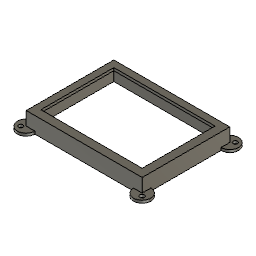
FullBoxDispenser_Assembly (Autodesk Fusion 360 archive; units mm, degrees)
design "BasicBreadboardHolder"
part number: 2026-05-25-11-22-07-482
Autodesk Fusion 360 part; units mm, degrees
note: some values were not read from the file. Set by a fixed rule: which sketch regions a step uses.
sketch "Sketch1" plane through (0, 0, 0) normal (0, 0, 1) x (1, 0, 0)
  line L0 (0, 0) -> (82, 0)
  line L1 (82, 0) -> (82, 61)
  line L2 (82, 61) -> (0, 61)
  line L3 (0, 61) -> (0, 0)
  line L4 (-2, 63) -> (84, 63)
  line L5 (84, 63) -> (84, -2)
  line L6 (84, -2) -> (-2, -2)
  line L7 (-2, -2) -> (-2, 63)
  circle A0 centre (-2, -2) radius 6.5
  circle A1 centre (-2, 63) radius 6.5
  circle A2 centre (84, 63) radius 6.5
  circle A3 centre (84, -2) radius 6.5
  circle A4 centre (-4, -4) radius 1.65
  circle A5 centre (-4, 65) radius 1.65
  circle A6 centre (86, 65) radius 1.65
  circle A7 centre (86, -4) radius 1.65
  line L8 (3, 58) -> (78, 58)
  line L9 (78, 58) -> (78, 4)
  line L10 (78, 4) -> (3, 4)
  line L11 (3, 4) -> (3, 58)
  dimension "d1" = 61
  dimension "d2" = 82
  dimension "d3" = 2
  dimension "d4" = 2
  dimension "d5" = 2
  dimension "d6" = 2
  dimension "d7" = 13
  dimension "d8" = 13
  dimension "d9" = 13
  dimension "d10" = 13
  dimension "d11" = 3.3
  dimension "d12" = 2
  dimension "d13" = 2
  dimension "d14" = 3.3
  dimension "d15" = 2
  dimension "d16" = 2
  dimension "d17" = 3.3
  dimension "d18" = 2
  dimension "d19" = 2
  dimension "d20" = 3.3
  dimension "d21" = 2
  dimension "d22" = 2
  dimension "d23" = 3
  dimension "d24" = 4
  dimension "d25" = 3
  dimension "d26" = 4
  constraint horizontal L0
  constraint vertical L1
  constraint horizontal L2
  constraint vertical L3
  constraint coincident L0.start L3.end
  constraint horizontal L4
  constraint vertical L5
  constraint horizontal L6
  constraint vertical L7
  constraint coincident L6.end L7.start
  constraint coincident L4.start L7.end
  constraint coincident L4.end L5.start
  constraint coincident L5.end L6.start
  constraint horizontal L8
  constraint vertical L9
  constraint horizontal L10
  constraint vertical L11
  measures "d1" distance of L0.start L2.end
  measures "d2" distance of L0.start L0.end
  measures "d3" distance of L2 L4
  measures "d4" distance of L1 L5
  measures "d5" distance of L3 L7
  measures "d6" distance of L0 L6
  measures "d7" diameter of A0
  measures "d8" diameter of A1
  measures "d9" diameter of A2
  measures "d10" diameter of A3
  measures "d11" diameter of A4
  measures "d12" vertical distance of L6.end A4.centre
  measures "d13" horizontal distance of L6.end A4.centre
  measures "d14" diameter of A5
  measures "d15" vertical distance of L4.start A5.centre
  measures "d16" horizontal distance of L4.start A5.centre
  measures "d17" diameter of A6
  measures "d18" horizontal distance of L4.end A6.centre
  measures "d19" vertical distance of L4.end A6.centre
  measures "d20" diameter of A7
  measures "d21" horizontal distance of L5.end A7.centre
  measures "d22" vertical distance of L5.end A7.centre
  measures "d23" distance of L2 L8
  measures "d24" distance of L0 L10
  measures "d25" distance of L3 L11
  measures "d26" distance of L1 L9
extrude "Extrude1" add sketch "Sketch1" along normal blind 2 contours L6 L7 A0 | L5 L6 A3 | L4 L7 A1 | L4 L5 A2 makes body 1 at (85.5519, 61.1596, 2) makes body 2 at (85.5519, -0.1596, 0) makes body 3 at (-3.5519, 61.1596, 0) makes body 4 at (-3.5519, -0.1596, 0)
extrude "Extrude2" add sketch "Sketch1" along normal blind 10 contours L0 L3 L6 L7 A0 | L0 L6 A0 A3 | L3 L7 A0 A1 | L0 L1 L5 L6 A3 | L2 L3 L4 L7 A1 | L1 L5 A2 A3 | L2 L4 A1 A2 | L1 L2 L4 L5 A2 bodies 1 2 3 4
extrude "Extrude3" add sketch "Sketch1" along normal blind 2 from surface at 10 contours L0 L3 A0 | L0 L3 L6 L7 A0 | L0 L1 L2 L3 A0 A1 A2 A3 | L0 L6 A0 A3 | L3 L7 A0 A1 | L0 L1 A3 | L0 L1 L5 L6 A3 | L2 L3 L4 L7 A1 | L2 L3 A1 | L1 L5 A2 A3 | L2 L4 A1 A2 | L1 L2 A2 | L1 L2 L4 L5 A2 bodies 1

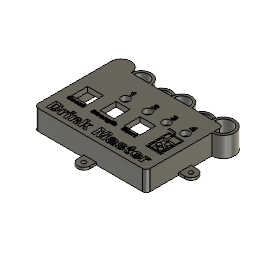
design "UIHolder"
part number: 2026-05-20-16-52-47-232
Autodesk Fusion 360 part; units mm, degrees
sketch "Sketch1" plane through (0, 0, 0) normal (0, 0, 1) x (1, 0, 0)
  line L0 (0, 0) -> (0, 57)
  line L1 (0, 0) -> (85, 0)
  line L2 (0, 57) -> (85, 57)
  line L3 (85, 57) -> (85, 0)
  line L4 (-2, 59) -> (87, 59)
  line L5 (87, 59) -> (87, -2)
  line L6 (87, -2) -> (-2, -2)
  line L7 (-2, -2) -> (-2, 59)
  circle A0 centre (6, 59) radius 6
  circle A1 centre (6, 59) radius 8
  line L8 (0, 59) -> (0, 57)
  line L9 (12, 59) -> (12, 57)
  circle A2 centre (77, 39) radius 3.25
  circle A3 centre (62, 39) radius 3.25
  circle A4 centre (47, 39) radius 3.25
  circle A5 centre (29.5, 39) radius 3.25
  line L10 (47.5, 32.5) -> (60, 32.5)
  line L11 (60, 32.5) -> (60, 20)
  line L12 (60, 20) -> (47.5, 20)
  line L13 (47.5, 20) -> (47.5, 32.5)
  line L14 (6, 20) -> (18.5, 20)
  line L15 (18.5, 20) -> (18.5, 32.5)
  line L16 (18.5, 32.5) -> (6, 32.5)
  line L17 (6, 32.5) -> (6, 20)
  line L18 (27.5, 33.5) -> (38.5, 33.5)
  line L19 (38.5, 33.5) -> (38.5, 21)
  line L20 (38.5, 21) -> (27.5, 21)
  line L21 (27.5, 21) -> (27.5, 33.5)
  circle A6 centre (22, 59) radius 8
  circle A7 centre (22, 59) radius 6
  circle A8 centre (38, 59) radius 8
  circle A9 centre (38, 59) radius 6
  circle A10 centre (54, 59) radius 8
  circle A11 centre (54, 59) radius 6
  circle A12 centre (70, 59) radius 8
  circle A13 centre (70, 59) radius 6
  circle A14 centre (87, 59) radius 9
  circle A15 centre (87, 59) radius 7
  circle A16 centre (-7, 28.5) radius 1.65
  circle A17 centre (42.5, -7) radius 1.65
  circle A18 centre (92, 28.5) radius 1.65
  line L22 (-2, 23.5) -> (-12, 23.5)
  line L23 (-12, 23.5) -> (-12, 33.5)
  line L24 (-12, 33.5) -> (-2, 33.5)
  line L25 (-2, 33.5) -> (-2, 23.5)
  line L26 (-2, 23.5) -> (-12, 33.5) construction
  line L27 (-12, 23.5) -> (-2, 33.5) construction
  line L28 (47.5, -2) -> (37.5, -2)
  line L29 (37.5, -2) -> (37.5, -12)
  line L30 (37.5, -12) -> (47.5, -12)
  line L31 (47.5, -12) -> (47.5, -2)
  line L32 (47.5, -2) -> (37.5, -12) construction
  line L33 (37.5, -2) -> (47.5, -12) construction
  line L34 (87, 23.5) -> (97, 23.5)
  line L35 (97, 23.5) -> (97, 33.5)
  line L36 (97, 33.5) -> (87, 33.5)
  line L37 (87, 33.5) -> (87, 23.5)
  line L38 (87, 23.5) -> (97, 33.5) construction
  line L39 (97, 23.5) -> (87, 33.5) construction
  point P0 (-7, 28.5)
  point P1 (42.5, -7)
  point P2 (92, 28.5)
  dimension "d1" = 57
  dimension "d2" = 85
  dimension "d3" = 85
  dimension "d4" = 2
  dimension "d5" = 2
  dimension "d6" = 2
  dimension "d7" = 2
  dimension "d8" = 12
  dimension "d9" = 8
  dimension "d12" = 6.5
  dimension "d13" = 8
  dimension "d15" = 6.5
  dimension "d17" = 15
  dimension "d18" = 6.5
  dimension "d20" = 15
  dimension "d21" = 6.5
  dimension "d22" = 18
  dimension "d23" = 18
  dimension "d24" = 18
  dimension "d25" = 18
  dimension "d26" = 17.5
  dimension "d27" = 12.5
  dimension "d28" = 12.5
  dimension "d29" = 25
  dimension "d30" = 20
  dimension "d31" = 12.5
  dimension "d32" = 12.5
  dimension "d33" = 20
  dimension "d34" = 6
  dimension "d35" = 12.5
  dimension "d36" = 11
  dimension "d37" = 9
  dimension "d38" = 21
  dimension "d42" = 16
  dimension "d43" = 12
  dimension "d44" = 16
  dimension "d45" = 12
  dimension "d46" = 16
  dimension "d47" = 12
  dimension "d48" = 16
  dimension "d49" = 12
  dimension "d50" = 14
  dimension "d75" = 3.3
  dimension "d76" = 3.3
  dimension "d77" = 3.3
  dimension "d78" = 30.5
  dimension "d79" = 30.5
  dimension "d80" = 44.5
  dimension "d81" = 5
  dimension "d82" = 5
  dimension "d83" = 5
  dimension "d84" = 10
  dimension "d85" = 10
  dimension "d86" = 10
  dimension "d87" = 10
  dimension "d88" = 10
  dimension "d89" = 10
  constraint coincident L0.start L1.start
  constraint vertical L0
  constraint perpendicular L0 L1
  constraint perpendicular L0 L2
  constraint horizontal L4
  constraint vertical L5
  constraint horizontal L6
  constraint vertical L7
  constraint coincident L4 A0.centre
  constraint concentric A0 A1
  constraint coincident L4.start A1
  constraint coincident A0 L8.start
  constraint coincident L4 L8.start
  constraint coincident L4 L9.start
  constraint coincident A0 L9.start
  constraint coincident L2 L9.end
  constraint perpendicular L2 L9
  constraint horizontal L10
  constraint vertical L11
  constraint horizontal L12
  constraint vertical L13
  constraint horizontal L14
  constraint vertical L15
  constraint horizontal L16
  constraint vertical L17
  constraint horizontal L18
  constraint vertical L19
  constraint horizontal L20
  constraint vertical L21
  constraint coincident L4 A6.centre
  constraint tangent A1 A6
  constraint concentric A6 A7
  constraint coincident L4 A8.centre
  constraint tangent A6 A8
  constraint concentric A8 A9
  constraint coincident L4 A10.centre
  constraint tangent A8 A10
  constraint concentric A10 A11
  constraint coincident L4 A12.centre
  constraint tangent A10 A12
  constraint concentric A12 A13
  constraint coincident L4.end L5.start
  constraint tangent A12 A14
  constraint concentric A14 A15
  constraint horizontal L22
  constraint perpendicular L22 L23
  constraint parallel L22 L24
  constraint parallel L23 L25
  constraint coincident L26 P0
  constraint coincident L27 P0
  constraint coincident P0 A16.centre
  constraint horizontal L28
  constraint perpendicular L28 L29
  constraint parallel L28 L30
  constraint parallel L29 L31
  constraint coincident L32 P1
  constraint coincident L33 P1
  constraint coincident P1 A17.centre
  constraint horizontal L34
  constraint perpendicular L34 L35
  constraint parallel L34 L36
  constraint parallel L35 L37
  constraint coincident L38 P2
  constraint coincident L39 P2
  constraint coincident P2 A18.centre
  measures "d1" distance of L0.start L0.end
  measures "d2" distance of L0.start L1.end
  measures "d3" distance of L0.end L2.end
  measures "d4" distance of L2 L4
  measures "d5" distance of L0 L7
  measures "d6" distance of L1 L6
  measures "d7" distance of L3 L5
  measures "d8" diameter of A0
  measures "d9" distance of L4.start A0.centre
  measures "d12" diameter of A2
  measures "d13" distance of L3 A2.centre
  measures "d15" diameter of A3
  measures "d17" distance of A2.centre A3.centre
  measures "d18" diameter of A4
  measures "d20" distance of A3.centre A4.centre
  measures "d21" diameter of A5
  measures "d22" distance of L2 A5.centre
  measures "d23" distance of L2 A4.centre
  measures "d24" distance of L2 A3.centre
  measures "d25" distance of L2 A2.centre
  measures "d26" distance of A4.centre A5.centre
  measures "d27" distance of L10.start L10.end
  measures "d28" distance of L10.start L12.end
  measures "d29" distance of L3 L11
  measures "d30" distance of L1 L12
  measures "d31" distance of L15.end L16.end
  measures "d32" distance of L14.end L15.end
  measures "d33" distance of L1 L14
  measures "d34" distance of L0 L17
  measures "d35" distance of L18.start L20.end
  measures "d36" distance of L18.start L18.end
  measures "d37" distance of L13 L19
  measures "d38" distance of L1 L20
  measures "d42" diameter of A6
  measures "d43" diameter of A7
  measures "d44" diameter of A8
  measures "d45" diameter of A9
  measures "d46" diameter of A10
  measures "d47" diameter of A11
  measures "d48" diameter of A12
  measures "d49" diameter of A13
  measures "d50" diameter of A15
  measures "d75" diameter of A16
  measures "d76" diameter of A17
  measures "d77" diameter of A18
  measures "d78" vertical distance of L4.start P0
  measures "d79" vertical distance of L4.end P2
  measures "d80" horizontal distance of L5.end P1
  measures "d81" distance of L6 P1
  measures "d82" distance of L7 P0
  measures "d83" distance of L5 P2
  measures "d84" distance of L22.end L23.end
  measures "d85" distance of L22.start L22.end
  measures "d86" distance of L29.end L30.end
  measures "d87" distance of L28.start L30.end
  measures "d88" distance of L34.end L35.end
  measures "d89" distance of L35.end L36.end
extrude "Extrude4" add sketch "Sketch1" along normal blind 2 contours L7 L22 L23 L24 L25 | L5 L34 L35 L36 L37 | L6 L28 L29 L30 L31 makes body 1 at (-7.0411, 24.6182, 0) makes body 2 at (42.5411, -3.1182, 0) makes body 3 at (91.9589, 24.6182, 0)
fillet "Fillet4" radius 5 6 edges at (-12, 23.5, 1) (-12, 33.5, 1) (37.5, -12, 1) (47.5, -12, 1) (97, 23.5, 1) (97, 33.5, 1) on bodies 1 2 3
extrude "Extrude1" add sketch "Sketch1" along normal blind 12 contours L0 L1 L3 L5 L6 L7 A1 A14 L25 L28 L37 | L0 L4 A1 L8 | L4 A0 A1 | L2 A1 A6 | L2 L4 A1 L9 | L3 L5 A14 A15 | L4 A6 A7 | L2 L4 A6 A7 | L2 L3 L4 L5 A15 | L2 L4 A14 A15 | L2 A12 A14 | L4 L5 A14 A15 | L2 L4 A7 | L2 L4 A6 A7 | L4 A8 A9 | L2 A6 A8 | L2 L4 A8 A9 | L2 L4 A12 A13 | L4 A12 A13 | L2 L4 A9 | L2 L4 A8 A9 | L4 A10 A11 | L2 A8 A10 | L2 L4 A10 A11 | L2 L4 A13 | L2 L4 A12 A13 | L2 A10 A12 | L2 L4 A10 A11 | L2 L4 A11 bodies 1 2 3
extrude "Extrude2" add sketch "Sketch1" along normal blind 4 from surface at 12 contours L0 L1 L3 L5 L6 L7 A1 A14 L25 L28 L37 | L0 L1 L2 L3 A1 A6 A8 A10 A12 A14 | L0 L4 A1 L8 | L0 L2 A0 A1 | L2 A0 L8 | L4 A0 A1 | L2 A1 A6 | L2 L4 A1 L9 | L2 L3 A14 A15 | L3 L5 A14 A15 | L2 L4 A0 | L2 A0 | L4 A0 | L4 A6 A7 | L2 L4 A6 A7 | L2 A0 L9 | L2 A6 A7 | L2 L3 A15 | L2 L3 L4 L5 A15 | L2 L4 A14 A15 | L2 A12 A14 | L4 L5 A14 A15 | L2 L4 A7 | L2 L4 A6 A7 | L2 A6 A8 | L2 L4 A8 A9 | L2 A7 | L2 A12 A13 | L2 L4 A12 A13 | L2 L4 A9 | L2 L4 A8 A9 | L4 A10 A11 | L2 A8 A10 | L2 L4 A10 A11 | L2 A8 A9 | L2 A13 | L2 L4 A13 | L2 L4 A12 A13 | L2 A10 A12 | L2 L4 A10 A11 | L2 A9 | L2 L4 A11 | L2 A10 A11 | L2 A11 bodies 1
fillet "Fillet3" radius 3 7 edges at (85, 57, 6) (87, 59, 8) (87, -2, 8) (85, 0, 6) (-2, -2, 8) (12, 57, 6) (0, 0, 6) on bodies 1
sketch "Sketch2" plane through (0, 0, 16) normal (0, 0, 1) x (-1, 0, 0)
  line L0 (-60, -32.5) -> (-60, -20)
  line L1 (-60, -20) -> (-47.5, -20)
  line L2 (-47.5, -20) -> (-47.5, -32.5)
  line L3 (-47.5, -32.5) -> (-60, -32.5)
  circle A0 centre (-47, -39) radius 3.25
  line L4 (-18.5, -20) -> (-6, -20)
  line L5 (-6, -20) -> (-6, -32.5)
  line L6 (-6, -32.5) -> (-18.5, -32.5)
  line L7 (-18.5, -32.5) -> (-18.5, -20)
  line L8 (-60, -59) -> (-48, -59)
  arc A1 (-60, -59) -> (-48, -59) centre (-54, -59) ccw
  circle A2 centre (-29.5, -39) radius 3.25
  circle A3 centre (-77, -39) radius 3.25
  arc A4 (-87, -56) -> (-84, -59) centre (-84, -56) ccw
  line L9 (-84, -59) -> (-80, -59)
  arc A5 (-87, -52) -> (-80, -59) centre (-87, -59) ccw
  line L10 (-87, -52) -> (-87, -56)
  line L11 (-38.5, -33.5) -> (-38.5, -21)
  line L12 (-38.5, -21) -> (-27.5, -21)
  line L13 (-27.5, -21) -> (-27.5, -33.5)
  line L14 (-27.5, -33.5) -> (-38.5, -33.5)
  line L15 (-28, -59) -> (-16, -59)
  arc A6 (-28, -59) -> (-16, -59) centre (-22, -59) ccw
  circle A7 centre (-62, -39) radius 3.25
  arc A8 (2, -1) -> (-1, 2) centre (-1, -1) ccw
  line L16 (-1, 2) -> (-84, 2)
  arc A9 (-84, 2) -> (-87, -1) centre (-84, -1) ccw
  line L17 (-87, -1) -> (-87, -50)
  arc A10 (-87, -50) -> (-78, -59) centre (-87, -59) ccw
  line L18 (-78, -59) -> (-62, -59)
  arc A11 (-62, -59) -> (-46, -59) centre (-54, -59) ccw
  line L19 (-46, -59) -> (-30, -59)
  arc A12 (-30, -59) -> (-14, -59) centre (-22, -59) ccw
  arc A13 (-14, -59) -> (2, -59) centre (-6, -59) ccw
  line L20 (2, -59) -> (2, -1)
  line L21 (0, 5) -> (-85, 5) construction
  line L22 (-85, 5) -> (-85, -10) construction
  line L23 (-85, -10) -> (0, -10) construction
  line L24 (0, -10) -> (0, 5) construction
  line L25 (-80.7167, -33.0536) -> (-73.974, -33.0536)
  line L26 (-73.974, -33.0536) -> (-73.8798, -33.7934)
  spline S0 degree 3 poles (-73.8798, -33.7934) (-73.8174, -34.4845) (-73.2798, -35.8297) (-71.6997, -35.9736) knots 0 0 0 0 1 1 1 1
  spline S1 degree 3 poles (-71.6997, -35.9736) (-70.1704, -36.1122) (-67.2864, -36.2477) (-67.1637, -36.254) knots 0 0 0 0 1 1 1 1
  line L27 (-67.1637, -36.254) -> (-67.1118, -35.1386)
  spline S2 degree 3 poles (-67.1118, -35.1386) (-67.1414, -35.1375) (-70.0942, -34.9978) (-71.5991, -34.8613) knots 0 0 0 0 1 1 1 1
  spline S3 degree 3 poles (-71.5991, -34.8613) (-72.6236, -34.7681) (-72.7569, -33.7987) (-72.7707, -33.6728) knots 0 0 0 0 1 1 1 1
  line L28 (-72.7707, -33.6728) -> (-72.849, -33.0536)
  line L29 (-72.849, -33.0536) -> (-70.5768, -33.0536)
  line L30 (-70.5768, -33.0536) -> (-69.7396, -33.0536)
  line L31 (-69.7396, -33.0536) -> (-69.7396, -32.2165)
  line L32 (-69.7396, -32.2165) -> (-69.7396, -15.6684)
  line L33 (-69.7396, -15.6684) -> (-69.7396, -14.8313)
  line L34 (-69.7396, -14.8313) -> (-70.5768, -14.8313)
  line L35 (-70.5768, -14.8313) -> (-80.7177, -14.8313)
  line L36 (-80.7177, -14.8313) -> (-81.5549, -14.8313)
  line L37 (-81.5549, -14.8313) -> (-81.5549, -15.6684)
  line L38 (-81.5549, -15.6684) -> (-81.5549, -32.2165)
  line L39 (-81.5549, -32.2165) -> (-81.5549, -33.0536)
  line L40 (-81.5549, -33.0536) -> (-80.7167, -33.0536)
  line L41 (-80.7167, -15.6684) -> (-70.5768, -15.6684)
  line L42 (-70.5768, -15.6684) -> (-70.5768, -32.2165)
  line L43 (-70.5768, -32.2165) -> (-72.9549, -32.2165)
  line L44 (-72.9549, -32.2165) -> (-73.5316, -27.6583)
  line L45 (-73.5316, -27.6583) -> (-71.1356, -27.6583)
  line L46 (-71.1356, -27.6583) -> (-71.1356, -16.2272)
  line L47 (-71.1356, -16.2272) -> (-80.1589, -16.2272)
  line L48 (-80.1589, -16.2272) -> (-80.1589, -27.6572)
  line L49 (-80.1589, -27.6572) -> (-74.6577, -27.6572)
  line L50 (-74.6577, -27.6572) -> (-74.0799, -32.2165)
  line L51 (-74.0799, -32.2165) -> (-80.7167, -32.2165)
  line L52 (-80.7167, -32.2165) -> (-80.7167, -15.6684)
  spline S4 degree 3 poles (-75.2059, -22.4015) (-75.498, -22.2967) (-75.6504, -21.975) (-75.5467, -21.6829) knots 0 0 0 0 1 1 1 1
  line L53 (-75.5467, -21.6829) -> (-74.9085, -19.8943)
  spline S5 degree 3 poles (-74.9085, -19.8943) (-74.8038, -19.6022) (-74.482, -19.4488) (-74.1899, -19.5535) knots 0 0 0 0 1 1 1 1
  line L54 (-74.1899, -19.5535) -> (-72.4013, -20.1917)
  spline S6 degree 3 poles (-72.4013, -20.1917) (-72.1082, -20.2965) (-71.9558, -20.6172) (-72.0606, -20.9103) knots 0 0 0 0 1 1 1 1
  line L55 (-72.0606, -20.9103) -> (-72.6977, -22.6989)
  spline S7 degree 3 poles (-72.6977, -22.6989) (-72.8025, -22.991) (-73.1242, -23.1434) (-73.4163, -23.0397) knots 0 0 0 0 1 1 1 1
  line L56 (-73.4163, -23.0397) -> (-75.2059, -22.4015)
  line L57 (-79.216, -25.0854) -> (-78.5778, -23.2969)
  spline S8 degree 3 poles (-78.5778, -23.2969) (-78.473, -23.0048) (-78.1513, -22.8513) (-77.8592, -22.9571) knots 0 0 0 0 1 1 1 1
  line L58 (-77.8592, -22.9571) -> (-76.0706, -23.5943)
  spline S9 degree 3 poles (-76.0706, -23.5943) (-75.7785, -23.699) (-75.625, -24.0197) (-75.7309, -24.3129) knots 0 0 0 0 1 1 1 1
  line L59 (-75.7309, -24.3129) -> (-76.368, -26.1014)
  spline S10 degree 3 poles (-76.368, -26.1014) (-76.4738, -26.3946) (-76.7934, -26.547) (-77.0866, -26.4422) knots 0 0 0 0 1 1 1 1
  line L60 (-77.0866, -26.4422) -> (-78.8752, -25.8051)
  spline S11 degree 3 poles (-78.8752, -25.8051) (-79.1662, -25.6993) (-79.3197, -25.3775) (-79.216, -25.0854) knots 0 0 0 0 1 1 1 1
  spline S12 degree 3 poles (-79.4869, -18.4) (-79.5948, -18.11) (-79.4456, -17.7851) (-79.1546, -17.6771) knots 0 0 0 0 1 1 1 1
  line L61 (-79.1546, -17.6771) -> (-77.3723, -17.0188)
  spline S13 degree 3 poles (-77.3723, -17.0188) (-77.0824, -16.9098) (-76.7585, -17.0601) (-76.6506, -17.3501) knots 0 0 0 0 1 1 1 1
  line L62 (-76.6506, -17.3501) -> (-75.9912, -19.1323)
  spline S14 degree 3 poles (-75.9912, -19.1323) (-75.8833, -19.4234) (-76.0325, -19.7462) (-76.3235, -19.8552) knots 0 0 0 0 1 1 1 1
  line L63 (-76.3235, -19.8552) -> (-78.1058, -20.5134)
  spline S15 degree 3 poles (-78.1058, -20.5134) (-78.3957, -20.6214) (-78.7196, -20.4722) (-78.8275, -20.1811) knots 0 0 0 0 1 1 1 1
  line L64 (-78.8275, -20.1811) -> (-79.4869, -18.4)
  line L65 (-23.8535, -40.2294) -> (-33.8535, -40.2294) construction
  line L66 (-33.8535, -40.2294) -> (-33.8535, -47.2294) construction
  line L67 (-33.8535, -47.2294) -> (-23.8535, -47.2294) construction
  line L68 (-23.8535, -47.2294) -> (-23.8535, -40.2294) construction
  line L69 (-42.0223, -40.2294) -> (-52.0223, -40.2294) construction
  line L70 (-52.0223, -40.2294) -> (-52.0223, -47.2294) construction
  line L71 (-52.0223, -47.2294) -> (-42.0223, -47.2294) construction
  line L72 (-42.0223, -47.2294) -> (-42.0223, -40.2294) construction
  line L73 (-57.0223, -40.2294) -> (-67.0223, -40.2294) construction
  line L74 (-67.0223, -40.2294) -> (-67.0223, -47.2294) construction
  line L75 (-67.0223, -47.2294) -> (-57.0223, -47.2294) construction
  line L76 (-57.0223, -47.2294) -> (-57.0223, -40.2294) construction
  line L77 (-72.0223, -40.2294) -> (-82.0223, -40.2294) construction
  line L78 (-82.0223, -40.2294) -> (-82.0223, -47.2294) construction
  line L79 (-82.0223, -47.2294) -> (-72.0223, -47.2294) construction
  line L80 (-72.0223, -47.2294) -> (-72.0223, -40.2294) construction
  line L81 (-6.9491, -12.274) -> (-16.9491, -12.274) construction
  line L82 (-16.9491, -12.274) -> (-16.9491, -19.274) construction
  line L83 (-16.9491, -19.274) -> (-6.9491, -19.274) construction
  line L84 (-6.9491, -19.274) -> (-6.9491, -12.274) construction
  line L85 (-28.9491, -12.274) -> (-38.9491, -12.274) construction
  line L86 (-38.9491, -12.274) -> (-38.9491, -19.274) construction
  line L87 (-38.9491, -19.274) -> (-28.9491, -19.274) construction
  line L88 (-28.9491, -19.274) -> (-28.9491, -12.274) construction
  line L89 (-48.8026, -12.3696) -> (-58.8026, -12.3696) construction
  line L90 (-58.8026, -12.3696) -> (-58.8026, -19.3696) construction
  line L91 (-58.8026, -19.3696) -> (-48.8026, -19.3696) construction
  line L92 (-48.8026, -19.3696) -> (-48.8026, -12.3696) construction
  dimension "d57" = 8
  dimension "d59" = 4
  dimension "d60" = 0
  dimension "d61" = 4
  dimension "d62" = 0
  dimension "d63" = 4
  dimension "d64" = 0
  dimension "d65" = 4
  dimension "d66" = 0
  dimension "d67" = 3
  dimension "d69" = 3
  dimension "d71" = 3
  text T0 "Drink Master" font "Arial Black" height 8 align centre top in box 85 x 15 at (0, 5) x (-1, 0) y (0, -1) spacing 1
  text T1 "1" font "Arial Black" height 4 align centre top in box 10 x 7 at (-23.8535, -40.2294) x (-1, 0) y (0, -1) spacing 1
  text T2 "2" font "Arial Black" height 4 align centre top in box 10 x 7 at (-42.0223, -40.2294) x (-1, 0) y (0, -1) spacing 1
  text T3 "3" font "Arial Black" height 4 align centre top in box 10 x 7 at (-57.0223, -40.2294) x (-1, 0) y (0, -1) spacing 1
  text T4 "4" font "Arial Black" height 4 align centre top in box 10 x 7 at (-72.0223, -40.2294) x (-1, 0) y (0, -1) spacing 1
  text T5 "Count" font "Arial Black" height 3 align centre top in box 10 x 7 at (-6.9491, -12.274) x (-1, 0) y (0, -1) spacing 1
  text T6 "Strength" font "Arial Black" height 3 align centre top in box 10 x 7 at (-28.9491, -12.274) x (-1, 0) y (0, -1) spacing 1
  text T7 "Start" font "Arial Black" height 3 align centre top in box 10 x 7 at (-48.8026, -12.3696) x (-1, 0) y (0, -1) spacing 1
extrude "Extrude3" cut sketch "Sketch2" sketch "Sketch2" against normal blind 2 contours L25 L26 S0 S1 L27 S2 S3 L28 L29 L30 L31 L32 L33 L34 L35 L36 L37 L38 L39 L40 of sketch 2 text T2 T1 T3 T4 T0 T7 T6 T5 bodies 1
equation "d58 = 'Drink Master'"
equation "d60 = '1'"
equation "d62 = '2'"
equation "d64 = '3'"
equation "d66 = '4'"
equation "d68 = 'Count'"
equation "d70 = 'Strength'"
equation "d72 = 'Start'"

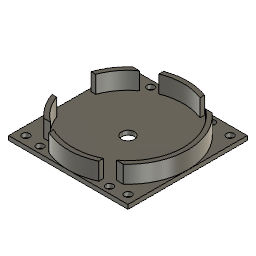
design "Box dispenser (Assembly)"
part number: 2026-05-20-10-56-44-048
Autodesk Fusion 360 part; units mm, degrees
sketch "Sketch1" plane through (0, 0, 0) normal (0, 0, 1) x (1, 0, 0)
  line L0 (0, 55) -> (0, 0)
  circle A0 centre (51, 51) radius 1.65
  circle A1 centre (4, 51) radius 1.65
  line L1 (25, 0) -> (30, 0)
  line L2 (0, 0) -> (55, 0)
  line L3 (55, 55) -> (0, 55)
  circle A2 centre (4, 4) radius 1.65
  circle A3 centre (51, 4) radius 1.65
  line L4 (55, 0) -> (55, 55)
  line L5 (45, 55) -> (9.9854, 55)
  line L6 (45, 55) -> (38, 55)
  circle A4 centre (11.5, 3) radius 1.65
  line L7 (16.9854, 55) -> (9.9854, 55)
  circle A5 centre (43.5, 3) radius 1.65
  line L8 (8, 0) -> (47, 0)
  circle A6 centre (13.4854, 52) radius 1.65
  circle A7 centre (41.5, 52) radius 1.65
  circle A8 centre (27.5, 27.5) radius 3
  point P0 (45, 45)
  dimension "d30" = 3.3
  dimension "d31" = 4
  dimension "d32" = 4
  dimension "d33" = 3.3
  dimension "d34" = 4
  dimension "d35" = 4
  dimension "d36" = 3.3
  dimension "d37" = 4
  dimension "d38" = 4
  dimension "d39" = 3.3
  dimension "d40" = 4
  dimension "d41" = 4
  dimension "d55" = 3.3
  dimension "d56" = 3.3
  dimension "d57" = 3
  dimension "d59" = 3
  dimension "d60" = 3.3
  dimension "d61" = 3.3
  dimension "d62" = 3
  dimension "d65" = 3
  dimension "d69" = 6
  dimension "d70" = 55
  dimension "d71" = 27.5
  dimension "d72" = 55
  dimension "d73" = 27.5
  constraint horizontal L2
  constraint vertical L4
  constraint horizontal L3
  constraint vertical L0
  constraint horizontal L1
  constraint coincident L1.start L2
  constraint coincident L5.start L6.start
  constraint coincident L5.end L7.end
  measures "d30" diameter of A2
  measures "d31" distance of A2.centre L2
  measures "d32" distance of A2.centre L0
  measures "d33" diameter of A3
  measures "d34" distance of A3.centre L2
  measures "d35" distance of A3.centre L4
  measures "d36" diameter of A1
  measures "d37" distance of A1.centre L3
  measures "d38" distance of A1.centre L0
  measures "d39" diameter of A0
  measures "d40" distance of A0.centre L3
  measures "d41" distance of A0.centre L4
  measures "d55" diameter of A7
  measures "d56" diameter of A6
  measures "d57" distance of A7.centre L5
  measures "d59" distance of A6.centre L5
  measures "d60" diameter of A5
  measures "d61" diameter of A4
  measures "d62" distance of A5.centre L8
  measures "d65" distance of A4.centre L8
  measures "d69" diameter of A8
  measures "d70" distance of L0.start L0.end
  measures "d71" distance of L3 A8.centre
  measures "d72" distance of L0.start L3.start
  measures "d73" distance of L4 A8.centre
extrude "Extrude1" add sketch "Sketch1" along normal blind 2
sketch "Sketch2" plane through (0, 0, 2) normal (0, 0, 1) x (-1, 0, 0)
  line L0 (0, 0) -> (-55, 0)
  line L1 (-55, 0) -> (-55, -55)
  line L2 (-55, -55) -> (0, -55)
  line L3 (0, -55) -> (0, 0)
  circle A0 centre (-51, -51) radius 1.65
  circle A1 centre (-4, -51) radius 1.65
  circle A2 centre (-51, -4) radius 1.65
  circle A3 centre (-13.4854, -52) radius 1.65
  circle A4 centre (-43.5, -3) radius 1.65
  circle A5 centre (-4, -4) radius 1.65
  circle A6 centre (-41.5, -52) radius 1.65
  circle A7 centre (-11.5, -3) radius 1.65
  circle A8 centre (-27.5, -27.5) radius 3
  circle A9 centre (-27.5, -27.5) radius 27.5
  circle A10 centre (-27.5, -27.5) radius 25.5
  line L4 (-18, -48) -> (-8.9708, -48)
  line L5 (-8.9708, -48) -> (-8.9708, -56)
  line L6 (-8.9708, -56) -> (-18, -56)
  line L7 (-18, -56) -> (-18, -48)
  line L8 (-18, -48) -> (-8.9708, -56) construction
  line L9 (-8.9708, -48) -> (-18, -56) construction
  line L10 (-37, -48) -> (-46, -48)
  line L11 (-46, -48) -> (-46, -56)
  line L12 (-46, -56) -> (-37, -56)
  line L13 (-37, -56) -> (-37, -48)
  line L14 (-37, -48) -> (-46, -56) construction
  line L15 (-46, -48) -> (-37, -56) construction
  line L16 (-39, -7) -> (-48, -7)
  line L17 (-48, -7) -> (-48, 1)
  line L18 (-48, 1) -> (-39, 1)
  line L19 (-39, 1) -> (-39, -7)
  line L20 (-39, -7) -> (-48, 1) construction
  line L21 (-48, -7) -> (-39, 1) construction
  line L22 (-16, -7) -> (-7, -7)
  line L23 (-7, -7) -> (-7, 1)
  line L24 (-7, 1) -> (-16, 1)
  line L25 (-16, 1) -> (-16, -7)
  line L26 (-16, -7) -> (-7, 1) construction
  line L27 (-7, -7) -> (-16, 1) construction
  line L28 (0, -36.5) -> (-10, -36.5)
  line L29 (-10, -36.5) -> (-10, -18.5)
  line L30 (-10, -18.5) -> (0, -18.5)
  line L31 (0, -18.5) -> (0, -36.5)
  point P0 (-13.4854, -52)
  point P1 (-41.5, -52)
  point P2 (-43.5, -3)
  point P3 (-11.5, -3)
  dimension "d74" = 2
  dimension "d75" = 51
  dimension "d78" = 18
  dimension "d79" = 18.5
  constraint concentric A8 A9
  constraint concentric A8 A10
  constraint horizontal L4
  constraint perpendicular L4 L5
  constraint parallel L4 L6
  constraint parallel L5 L7
  constraint coincident L8 P0
  constraint coincident L9 P0
  constraint coincident P0 A3.centre
  constraint horizontal L10
  constraint perpendicular L10 L11
  constraint parallel L10 L12
  constraint parallel L11 L13
  constraint coincident L14 P1
  constraint coincident L15 P1
  constraint coincident P1 A6.centre
  constraint horizontal L16
  constraint perpendicular L16 L17
  constraint parallel L16 L18
  constraint parallel L17 L19
  constraint coincident L20 P2
  constraint coincident L21 P2
  constraint coincident P2 A4.centre
  constraint horizontal L22
  constraint perpendicular L22 L23
  constraint parallel L22 L24
  constraint parallel L23 L25
  constraint coincident L26 P3
  constraint coincident L27 P3
  constraint coincident P3 A7.centre
  constraint horizontal L28
  constraint vertical L29
  constraint horizontal L30
  constraint vertical L31
  constraint coincident L3 L28.start
  measures "d74" distance of A9 A10
  measures "d75" diameter of A10
  measures "d78" distance of L28.end L29.end
  measures "d79" distance of L2.end L28.start
extrude "Extrude2" add sketch "Sketch2" along normal blind 8 contours A9 A10 L22 L30 | A9 A10 L19 L25 | A9 A10 L4 L28 | A9 A10 L10 L16 | A9 A10 L7 L13

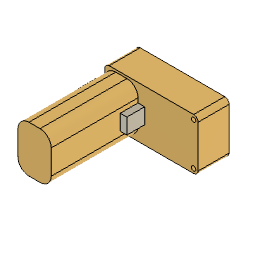
design "DC Motor from Hanka Dubovská"
part number: 2026-01-29-20-00-23-988
Autodesk Fusion 360 part; units mm, degrees
sketch "Sketch1" plane through (0, 0, 0) normal (0, 0, 1) x (1, 0, 0)
  line L0 (0, 0) -> (42, 0)
  line L1 (42, 0) -> (42, 14)
  line L2 (42, 14) -> (0, 14)
  line L3 (0, 14) -> (0, 0)
  line L4 (0, 0) -> (20, 0)
  dimension "d1" = 42
  dimension "d2" = 14
  constraint horizontal L0
  constraint vertical L1
  constraint horizontal L2
  constraint vertical L3
  constraint coincident L0.start L3.end
  constraint horizontal L4
  measures "d1" distance of L1.end L2.end
  measures "d2" distance of L0.end L1.end
extrude "Extrude1" add sketch "Sketch1" along normal blind 23
extrude "Extrude2" add sketch "Sketch1" along normal blind 22
sketch "Sketch3" plane through (0, 0, 0) normal (0, 1, 0) x (1, 0, 0)
  line L0 (15, -1) -> (0, -1)
  line L1 (0, -1) -> (0, -22)
  line L2 (0, -22) -> (15, -22)
  line L3 (15, -22) -> (15, -1)
  dimension "d17" = 15
  constraint horizontal L0
  constraint vertical L1
  constraint horizontal L2
  constraint vertical L3
  measures "d17" distance of L1.end L2.end
extrude "Extrude4" add sketch "Sketch3" against normal blind 39
fillet "Fillet2" radius 5 4 edges at (0, -19.5, 22) (15, -19.5, 22) (0, -19.5, 1) (15, -19.5, 1)
fillet "Fillet3" radius 2 4 edges at (0, 7, 0) (42, 7, 0) (42, 7, 23) (0, 7, 23)
sketch "Sketch4" plane through (0, 0, 0) normal (-1, 0, 0) x (0, -1, 0)
  line L0 (0, 21) -> (-14, 21)
  line L1 (-14, 21) -> (-14, 2)
  line L2 (-14, 2) -> (0, 2)
  line L3 (0, 2) -> (0, 6)
  line L4 (0, 6) -> (39, 6)
  line L5 (39, 6) -> (39, 17)
  line L6 (39, 17) -> (0, 17)
  line L7 (0, 17) -> (0, 21)
  line L8 (0, 15) -> (8, 15)
  line L9 (8, 15) -> (8, 8)
  line L10 (8, 8) -> (0, 8)
  line L11 (0, 8) -> (0, 15)
  dimension "d20" = 8
  dimension "d21" = 7
  constraint horizontal L8
  constraint vertical L9
  constraint horizontal L10
  constraint vertical L11
  measures "d20" distance of L8.start L8.end
  measures "d21" distance of L8.start L10.end
extrude "Extrude5" add sketch "Sketch4" along normal blind 4 contours L8 L9 L10 L11
sketch "Sketch5" plane through (0, 14, 0) normal (0, 1, 0) x (-1, 0, 0)
  arc A0 (0, 21) -> (-2, 23) centre (-2, 21) ccw
  line L0 (-2, 23) -> (-40, 23)
  arc A1 (-40, 23) -> (-42, 21) centre (-40, 21) ccw
  line L1 (-42, 21) -> (-42, 2)
  arc A2 (-42, 2) -> (-40, 0) centre (-40, 2) ccw
  line L2 (-40, 0) -> (-2, 0)
  arc A3 (-2, 0) -> (0, 2) centre (-2, 2) ccw
  line L3 (0, 2) -> (0, 21)
  line L4 (-30.8362, 13.6553) -> (-29.8362, 13.6553)
  line L5 (-28.8362, 12.6553) -> (-28.8362, 9.6553)
  line L6 (-29.8362, 8.6553) -> (-30.8362, 8.6553)
  line L7 (-31.8362, 9.6553) -> (-31.8362, 12.6553)
  circle A4 centre (-21, 11.5403) radius 1.5
  arc A5 (-28.8362, 12.6553) -> (-29.8362, 13.6553) centre (-29.8362, 12.6553) ccw
  arc A6 (-30.8362, 13.6553) -> (-31.8362, 12.6553) centre (-30.8362, 12.6553) ccw
  arc A7 (-31.8362, 9.6553) -> (-30.8362, 8.6553) centre (-30.8362, 9.6553) ccw
  arc A8 (-29.8362, 8.6553) -> (-28.8362, 9.6553) centre (-29.8362, 9.6553) ccw
  point P0 (-28.8362, 13.6553)
  point P1 (-28.8362, 8.6553)
  point P2 (-31.8362, 8.6553)
  dimension "d24" = 3
  dimension "d25" = 5
  dimension "d26" = 3
  dimension "d37" = 1
  constraint horizontal L4
  constraint vertical L5
  constraint horizontal L6
  constraint vertical L7
  constraint coincident P0 L4
  constraint coincident P0 L5
  constraint tangent L4 A5
  constraint tangent L5 A5
  constraint tangent L4 A6
  constraint tangent L7 A6
  constraint equal A5 A6
  constraint coincident P2 L6
  constraint coincident P2 L7
  constraint tangent L6 A7
  constraint tangent L7 A7
  constraint equal A5 A7
  constraint coincident P1 L5
  constraint coincident P1 L6
  constraint tangent L5 A8
  constraint tangent L6 A8
  constraint equal A5 A8
  measures "d24" diameter of A4
  measures "d25" distance of P0 P1
  measures "d26" distance of P1 P2
  measures "d37" radius of A5
extrude "Extrude6" add sketch "Sketch5" along normal blind 8 contours L4 L5 L6 L7 A5 A6 A7 A8
sketch "Sketch6" plane through (0, 14, 0) normal (0, 1, 0) x (-1, 0, 0)
  circle A0 centre (-21, 11.5) radius 1.5
  dimension "d29" = 3
  measures "d29" diameter of A0
extrude "Extrude7" add sketch "Sketch6" along normal blind 1
sketch "Sketch7" plane through (15, 0, 0) normal (1, 0, 0) x (0, 1, 0)
  line L0 (-39, 6) -> (0, 6)
  line L1 (0, 6) -> (0, 17)
  line L2 (0, 17) -> (-39, 17)
  line L3 (-39, 17) -> (-39, 6)
  line L4 (0, 15) -> (-8, 15)
  line L5 (-8, 15) -> (-8, 8)
  line L6 (-8, 8) -> (0, 8)
  line L7 (0, 8) -> (0, 15)
  constraint horizontal L4
  constraint vertical L5
  constraint horizontal L6
  constraint vertical L7
  constraint coincident L1 L4.start
extrude "Extrude8" add sketch "Sketch7" along normal blind 3 contours L1 L4 L5 L6 L7
sketch "Sketch8" plane through (0, 14, 0) normal (0, 1, 0) x (-1, 0, 0)
  circle A0 centre (-21, 11.5) radius 1.5
  line L0 (-31.8362, 9.6553) -> (-31.8362, 12.6553)
  line L1 (-30.8362, 13.6553) -> (-29.8362, 13.6553)
  line L2 (-28.8362, 12.6553) -> (-28.8362, 9.6553)
  line L3 (-29.8362, 8.6553) -> (-30.8362, 8.6553)
  arc A1 (0, 21) -> (-2, 23) centre (-2, 21) ccw
  line L4 (-2, 23) -> (-40, 23)
  arc A2 (-40, 23) -> (-42, 21) centre (-40, 21) ccw
  line L5 (-42, 21) -> (-42, 2)
  arc A3 (-42, 2) -> (-40, 0) centre (-40, 2) ccw
  line L6 (-40, 0) -> (-2, 0)
  arc A4 (-2, 0) -> (0, 2) centre (-2, 2) ccw
  line L7 (0, 2) -> (0, 21)
  circle A5 centre (-40, 2) radius 1
  circle A6 centre (-40, 21) radius 1
  arc A7 (-30.8362, 13.6553) -> (-31.8362, 12.6553) centre (-30.8362, 12.6553) ccw
  arc A8 (-28.8362, 12.6553) -> (-29.8362, 13.6553) centre (-29.8362, 12.6553) ccw
  arc A9 (-29.8362, 8.6553) -> (-28.8362, 9.6553) centre (-29.8362, 9.6553) ccw
  arc A10 (-31.8362, 9.6553) -> (-30.8362, 8.6553) centre (-30.8362, 9.6553) ccw
  constraint concentric A3 A5
  constraint concentric A2 A6
hole "Hole1" at (40, 14, 2) at (40, 14, 21) direction (0, -1, 0) diameter 2 depth 14 tip angle 118

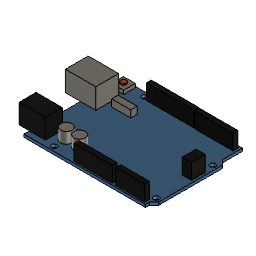
design "arduino"
part number: 2026-01-28-20-02-21-099
Autodesk Fusion 360 part; units mm, degrees
sketch "Sketch1" plane through (0, 0, 0) normal (0, 0, 1) x (1, 0, 0)
  line L0 (0, 0) -> (0, -52.8)
  line L1 (0, 0) -> (66, 0)
  line L2 (0, -52.8) -> (66, -52.8)
  line L3 (66, 0) -> (66, -10.9)
  line L4 (66, -52.8) -> (66, -50.7)
  line L5 (66, -50.7) -> (68.6, -48.1)
  line L6 (68.6, -48.1) -> (68.6, -13.5)
  line L7 (66, -10.9) -> (68.6, -13.5)
  circle A0 centre (15.3, -2.5) radius 1.5
  circle A1 centre (14, -50.3) radius 1.5
  circle A2 centre (66.1, -16.2) radius 1.5
  circle A3 centre (66.1, -46.9) radius 1.5
  line L8 (64.8, -1.3) -> (44, -1.3)
  line L9 (44, -1.3) -> (44, -3.9)
  line L10 (44, -3.9) -> (64.8, -3.9)
  line L11 (64.8, -3.9) -> (64.8, -1.3)
  line L12 (43.3, -1.1) -> (43.3, -3.7)
  line L13 (43.3, -3.7) -> (17.5, -3.7)
  line L14 (17.5, -3.7) -> (17.5, -1.1)
  line L15 (17.5, -1.1) -> (43.3, -1.1)
  line L16 (64.8, -51.9) -> (49.1, -51.9)
  line L17 (49.1, -51.9) -> (49.1, -49.3)
  line L18 (49.1, -49.3) -> (64.8, -49.3)
  line L19 (64.8, -49.3) -> (64.8, -51.9)
  line L20 (47.1, -51.9) -> (26.4, -51.9)
  line L21 (26.4, -51.9) -> (26.4, -49.3)
  line L22 (26.4, -49.3) -> (47.1, -49.3)
  line L23 (47.1, -49.3) -> (47.1, -51.9)
  line L24 (62.3, -21.5) -> (62.3, -29)
  line L25 (62.3, -29) -> (67.3, -29)
  line L26 (67.3, -29) -> (67.3, -21.5)
  line L27 (67.3, -21.5) -> (62.3, -21.5)
  line L28 (8.7, -49.8) -> (-5.6, -49.8)
  line L29 (-5.6, -49.8) -> (-5.6, -40.5)
  line L30 (-5.6, -40.5) -> (8.7, -40.5)
  line L31 (8.7, -40.5) -> (8.7, -49.8)
  line L32 (8.4, -9.6) -> (-8.2, -9.6)
  line L33 (-8.2, -9.6) -> (-8.2, -22.1)
  line L34 (-8.2, -22.1) -> (8.4, -22.1)
  line L35 (8.4, -22.1) -> (8.4, -9.6)
  line L36 (2, -0.6) -> (2, -7.1)
  line L37 (2, -7.1) -> (8.5, -7.1)
  line L38 (8.5, -7.1) -> (8.5, -0.6)
  line L39 (8.5, -0.6) -> (2, -0.6)
  line L40 (11.1, -12.7) -> (11.1, -16.2)
  line L41 (11.1, -16.2) -> (21.5, -16.2)
  line L42 (21.5, -16.2) -> (21.5, -12.7)
  line L43 (21.5, -12.7) -> (11.1, -12.7)
  circle A4 centre (14.2, -43.9) radius 3.1
  circle A5 centre (21.4, -43.9) radius 3.1
  circle A6 centre (5.1, -3.7) radius 1.475
  dimension "d1" = 52.8
  dimension "d2" = 66
  dimension "d3" = 66
  dimension "d4" = 10.9
  dimension "d5" = 2.1
  dimension "d6" = 135
  dimension "d7" = 135
  dimension "d8" = 2.6
  dimension "d9" = 2.6
  dimension "d10" = 3
  dimension "d11" = 15.3
  dimension "d12" = 2.5
  dimension "d13" = 3
  dimension "d14" = 14
  dimension "d15" = 2.5
  dimension "d16" = 3
  dimension "d17" = 2.5
  dimension "d18" = 16.2
  dimension "d19" = 3
  dimension "d20" = 2.5
  dimension "d21" = 5.9
  dimension "d22" = 2.6
  dimension "d23" = 20.8
  dimension "d24" = 1.3
  dimension "d25" = 1.2
  dimension "d26" = 2.6
  dimension "d27" = 25.8
  dimension "d28" = 17.5
  dimension "d29" = 1.1
  dimension "d30" = 2.6
  dimension "d31" = 15.7
  dimension "d32" = 1.2
  dimension "d33" = 0.9
  dimension "d34" = 2.6
  dimension "d35" = 20.7
  dimension "d37" = 0.9
  dimension "d38" = 2
  dimension "d39" = 7.5
  dimension "d40" = 5
  dimension "d41" = 1.3
  dimension "d42" = 17.6
  dimension "d43" = 9.3
  dimension "d44" = 14.3
  dimension "d45" = 5.6
  dimension "d46" = 3
  dimension "d47" = 12.5
  dimension "d48" = 16.6
  dimension "d49" = 8.2
  dimension "d50" = 9.6
  dimension "d51" = 6.5
  dimension "d52" = 6.5
  dimension "d53" = 2
  dimension "d54" = 0.6
  dimension "d55" = 3.5
  dimension "d56" = 10.4
  dimension "d57" = 12.7
  dimension "d58" = 2.7
  dimension "d59" = 6.2
  dimension "d60" = 5.5
  dimension "d61" = 8.9
  dimension "d62" = 6.2
  dimension "d63" = 8.9
  dimension "d64" = 7.2
  dimension "d73" = 2.95
  dimension "d74" = 3.1
  dimension "d75" = 3.1
  constraint coincident L0.start L1.start
  constraint vertical L0
  constraint perpendicular L0 L1
  constraint perpendicular L0 L2
  constraint perpendicular L1 L3
  constraint perpendicular L2 L4
  constraint parallel L4 L6
  constraint horizontal L8
  constraint perpendicular L8 L9
  constraint perpendicular L9 L10
  constraint perpendicular L8 L11
  constraint vertical L12
  constraint perpendicular L12 L13
  constraint perpendicular L13 L14
  constraint perpendicular L12 L15
  constraint horizontal L16
  constraint perpendicular L16 L17
  constraint perpendicular L17 L18
  constraint perpendicular L16 L19
  constraint parallel L2 L20
  constraint perpendicular L20 L21
  constraint perpendicular L21 L22
  constraint perpendicular L20 L23
  constraint vertical L24
  constraint perpendicular L24 L25
  constraint perpendicular L25 L26
  constraint perpendicular L24 L27
  constraint perpendicular L0 L28
  constraint perpendicular L28 L29
  constraint perpendicular L0 L30
  constraint perpendicular L28 L31
  constraint horizontal L32
  constraint perpendicular L32 L33
  constraint perpendicular L0 L34
  constraint perpendicular L32 L35
  constraint parallel L0 L36
  constraint perpendicular L0 L37
  constraint perpendicular L37 L38
  constraint perpendicular L36 L39
  constraint perpendicular L32 L40
  constraint perpendicular L0 L41
  constraint perpendicular L41 L42
  constraint perpendicular L40 L43
  measures "d1" distance of L0.start L0.end
  measures "d2" distance of L0.start L1.end
  measures "d3" distance of L0.end L2.end
  measures "d4" distance of L1.end L3.end
  measures "d5" distance of L2.end L4.end
  measures "d6" angle of L3 L7
  measures "d7" angle of L4 L5
  measures "d8" distance of L3 L6.end
  measures "d9" distance of L4 L5.end
  measures "d10" diameter of A0
  measures "d11" distance of L0 A0.centre
  measures "d12" distance of L1 A0.centre
  measures "d13" diameter of A1
  measures "d14" distance of L0 A1.centre
  measures "d15" distance of L2 A1.centre
  measures "d16" diameter of A2
  measures "d17" distance of L6 A2.centre
  measures "d18" distance of L1 A2.centre
  measures "d19" diameter of A3
  measures "d20" distance of L6 A3.centre
  measures "d21" distance of L2 A3.centre
  measures "d22" distance of L8 L10
  measures "d23" distance of L8.start L8.end
  measures "d24" distance of L1 L8
  measures "d25" distance of L3 L11
  measures "d26" distance of L12.start L12.end
  measures "d27" distance of L12.start L14.end
  measures "d28" distance of L0 L14
  measures "d29" distance of L1 L15
  measures "d30" distance of L16.start L18.end
  measures "d31" distance of L17.end L18.end
  measures "d32" distance of L4 L19
  measures "d33" distance of L2 L16
  measures "d34" distance of L20.end L21.end
  measures "d35" distance of L21.end L22.end
  measures "d37" distance of L2 L20
  measures "d38" distance of L17 L23
  measures "d39" distance of L24.start L24.end
  measures "d40" distance of L24.end L25.end
  measures "d41" distance of L6 L26
  measures "d42" distance of L10 L27
  measures "d43" distance of L28.end L29.end
  measures "d44" distance of L29.end L30.end
  measures "d45" distance of L0 L29
  measures "d46" distance of L2 L28
  measures "d47" distance of L32.end L33.end
  measures "d48" distance of L33.end L34.end
  measures "d49" distance of L0 L33
  measures "d50" distance of L1 L32
  measures "d51" distance of L36.start L38.end
  measures "d52" distance of L36.start L36.end
  measures "d53" distance of L0 L36
  measures "d54" distance of L1 L39
  measures "d55" distance of L41.end L42.end
  measures "d56" distance of L40.start L42.end
  measures "d57" distance of L1 L43
  measures "d58" distance of L35 L40
  measures "d59" diameter of A4
  measures "d60" distance of L31 A4.centre
  measures "d61" distance of L2 A4.centre
  measures "d62" diameter of A5
  measures "d63" distance of L2 A5.centre
  measures "d64" distance of A4.centre A5.centre
  measures "d73" diameter of A6
  measures "d74" distance of L39 A6.centre
  measures "d75" distance of L36 A6.centre
extrude "Extrude1" add sketch "Sketch1" along normal blind 1.6 contours L0 L1 L2 L3 L4 L5 L6 L7 L28 L30 L31 L32 L34 L35
extrude "Extrude2" add sketch "Sketch1" along normal blind 10 contours L8 L9 L10 L11 | L12 L13 L14 L15 | L16 L17 L18 L19 | L20 L21 L22 L23 | L24 L25 L26 L27
extrude "Extrude3" add sketch "Sketch1" along normal blind 7.6 contours A4 | A5
extrude "Extrude4" add sketch "Sketch1" along normal blind 5.4 contours L40 L41 L42 L43
extrude "Extrude5" add sketch "Sketch1" along normal blind 3.6 contours L36 L37 L38 L39
extrude "Extrude6" add sketch "Sketch1" along normal blind 4.3 contours A6
extrude "Extrude7" add sketch "Sketch1" along normal blind 12.7 contours L0 L32 L34 L35 | L0 L32 L33 L34
extrude "Extrude8" add sketch "Sketch1" along normal blind 12.3 contours L0 L28 L30 L31 | L0 L28 L29 L30
extrude "Extrude9" cut sketch "Sketch1" along normal blind 1.6 contours L0 L32 L33 L34 | L0 L28 L29 L30

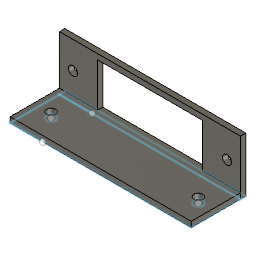
design "MotorHolderExtension"
part number: 2026-05-19-21-13-05-424
Autodesk Fusion 360 part; units mm, degrees
sketch "Sketch1" plane through (0, 0, 0) normal (0, 0, 1) x (1, 0, 0)
  line L0 (0, 18) -> (66.46, 18)
  line L1 (12, 18) -> (0, 18)
  line L2 (66.46, 18) -> (66.46, -0.0843)
  line L3 (0, -0.0843) -> (0, 18)
  line L4 (0, 0) -> (12, 0)
  circle A0 centre (6, 9) radius 1.65
  line L5 (0, 18) -> (0, 0)
  line L6 (66.46, -0.0843) -> (0, -0.0843)
  circle A1 centre (60, 9) radius 1.65
  line L7 (0, 18) -> (66.466, 18)
  line L8 (66.466, 18) -> (66.466, 20)
  line L9 (66.466, 20) -> (0, 20)
  line L10 (0, 20) -> (0, 18)
  dimension "d3" = 3.3
  dimension "d4" = 3.3
  dimension "d5" = 2
  constraint horizontal L0
  constraint vertical L2
  constraint horizontal L6
  constraint vertical L3
  constraint coincident L0.start L1.end
  constraint horizontal L7
  constraint vertical L8
  constraint horizontal L9
  constraint vertical L10
  measures "d3" diameter of A0
  measures "d4" diameter of A1
  measures "d5" distance of L0.start L9.end
extrude "Extrude1" add sketch "Sketch1" along normal blind 2 contours L0 L1 L2 L3 L5 L6 L7
extrude "Extrude2" add sketch "Sketch1" along normal blind 20 contours L0 L1 L7 L8 L9 L10
sketch "Sketch2" plane through (0, 18, 0) normal (0, -1, 0) x (1, 0, 0)
  line L0 (66.46, 2) -> (66.46, 0)
  line L1 (66.46, 0) -> (66.466, 0)
  line L2 (66.466, 0) -> (66.466, 20)
  line L3 (66.466, 20) -> (0, 20)
  line L4 (0, 20) -> (0, 2)
  line L5 (0, 2) -> (66.46, 2)
  line L6 (14, 2) -> (52.466, 2)
  line L7 (52.466, 2) -> (52.466, 18)
  line L8 (52.466, 18) -> (14, 18)
  line L9 (14, 18) -> (14, 2)
  circle A0 centre (61.466, 10) radius 1.65
  circle A1 centre (5, 10) radius 1.65
  dimension "d12" = 2
  dimension "d13" = 14
  dimension "d14" = 14
  dimension "d15" = 3.3
  dimension "d16" = 5
  dimension "d17" = 10
  dimension "d18" = 3.3
  dimension "d19" = 5
  dimension "d20" = 10
  constraint horizontal L6
  constraint vertical L7
  constraint horizontal L8
  constraint vertical L9
  constraint coincident L5 L6.start
  measures "d12" distance of L3 L8
  measures "d13" distance of L4 L9
  measures "d14" distance of L2 L7
  measures "d15" diameter of A0
  measures "d16" distance of L2 A0.centre
  measures "d17" distance of L3 A0.centre
  measures "d18" diameter of A1
  measures "d19" distance of L4 A1.centre
  measures "d20" distance of L3 A1.centre
extrude "Extrude3" cut sketch "Sketch2" against normal blind 2 contours L5 L6 L7 L8 L9 | A0 | A1
